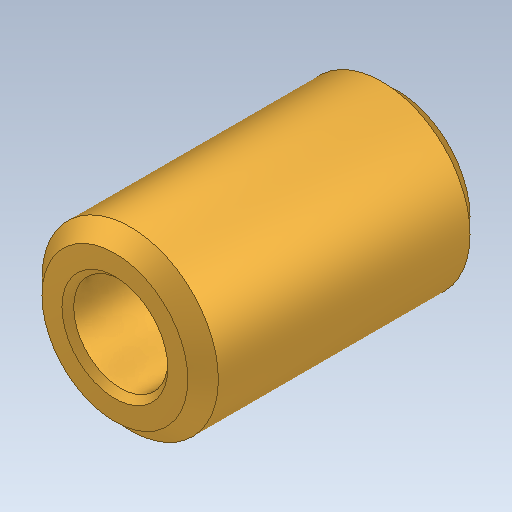
# Autodesk Inventor part: lm8uu-graphite
Saved by Autodesk Inventor 2020.4 (Build 244396000, 396)
## iProperties
Created: 2021-02-19
Part Number: lm8uu-graphite
Material: Brass, Soft Yellow
Document SubType Name: Modeling
Designer: AOB
Mass: 25.0136 g
Surface Area: 18.9682 cm^2
Volume: 2.9532 cm^3
Density: 8.47 g/cm^3
Appearance: Brass - Satin
Author: AOB
Autodesk Inventor part; units mm, degrees
ref_plane "YZ Plane" through (0, 0, 0) normal (1, 0, 0) x (0, 1, 0)
ref_plane "XZ Plane" through (0, 0, 0) normal (0, 1, 0) x (-1, 0, 0)
ref_plane "XY Plane" through (0, 0, 0) normal (0, 0, 1) x (1, 0, 0)
sketch "Sketch1" plane through (0, 0, 0) normal (0, 0, 1) x (1, 0, 0)
  circle A0 centre (0, 0) radius 4
  circle A1 centre (0, 0) radius 7.5
  dimension "d0" = 8
  dimension "d1" = 15
  constraints: 2 centre point, 2 coincident
  measures "d0" diameter of A0
  measures "d1" diameter of A1
extrude "Extrusion1" add sketch "Sketch1" along normal blind 24
chamfer "Chamfer1" distance 1.3 angle 45 2 edges at (-7.5, 0, 0) (-7.5, 0, 24)
chamfer "Chamfer2" distance 0.5 angle 45 1 edges at (-4, 0, 0)
chamfer "Chamfer3" distance 0.5 angle 45 1 edges at (-4, 0, 24)
body "Solid1"
